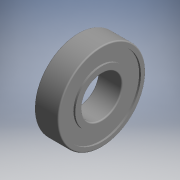
# Autodesk Inventor part: B6900ZZ
Saved by Autodesk Inventor 2017.3 (Build 213256000, 256)
## iProperties
Part Number: B6900ZZ
Material: Generic
Catalog Web Link: www.cadenas.de
Description: B6_ _ _ZZ, SB6_ _ _ZZ-Deep Groove Ball Bearings - Double Shield Type
Vendor: MISUMI
Document SubType Name: Modeling
Designer: partserver
Manufacturer: MISUMI
Mass: 1.66105 g
Surface Area: 12.7379 cm^2
Volume: 1.66105 cm^3
Density: 1 g/cm^3
Appearance: PSOLRGB-175-175-175
Category: PARTsolutions
Company: MISUMI
Title: B6900ZZ
Author: Cadenas PARTsolutions
Comments: Deep Groove Ball Bearings - Double Shield Type
PSOL_IDENT_0: {$CADENAS_DATA\23d-libs\misumi\metric\12_bearing_holders\sb6010zz.prj},171 {VTYP=3D},{NB=B6900ZZ},{L
PSOL_IDENT_1: INA=B6900ZZ},{NN=B6_ _ _ZZ, SB6_ _ _ZZ},{DATE=22.10.2019 07:39:52},{GEOMDATE=22.10.2019 06:26:04},{V
PSOL_IDENT_2: ERSION=},{LINEID=30},{WBVAR=TS},{WBNUMERIC=}  {NB=B6900ZZ},{LINA=B6900ZZ},{KT=DUMMY},{PN=B6900ZZ},{T
PSOL_IDENT_3: S=},{TS1= '', 'Steel', 'S', 'Stainless Steel'},{MAT=52100 Bearing Steel},{BN=6900ZZ},{DD=10},{D=22},
PSOL_IDENT_4: {B=6},{RR=0.3},{CR=2.70},{COR=1.27},{CRS=2.70},{CRSS=2.29},{CORS=1.27},{CORSS=1.02},{DD1=20.80},{R1=
PSOL_IDENT_5: 0.20},{R2=0.3},{DSMIN=12.0},{DSMAX=13.00},{DS1=13.00},{DDHH=20.0},{R=0.3},{MASS=9},{MASS11=9},{AA=5.
PSOL_IDENT_6: 1000},{BB=1.2000},{CC=1.7000},{TYS=w/o Retaining Ring}
NB: B6900ZZ
NN: B6_ _ _ZZ, SB6_ _ _ZZ
NT: Deep Groove Ball Bearings - Double Shield Type
NBSYN: $PN.
LINA: B6900ZZ
CATALOG: Misumi
PN: B6900ZZ
TS: Steel
MAT: 52100 Bearing Steel
BN: 6900ZZ
DD: 10
D: 22
B: 6
RR: 0.3
CR: 2.70
COR: 1.27
DSMIN: 12
DSMAX: 13
DDHH: 20
R: 0.3
MASS: 9
SUPPLIER: MISUMI
ARTICLENO: B6900ZZ
BOMINFO: B6900ZZ
CREATOR: CADENAS GmbH
Autodesk Inventor part; units mm, degrees
sketch "Sketch_1" plane through (0, 0, 0) normal (0, 0, 1) x (1, 0, 0)
  line L0 (6, 0) -> (0, 0)
  arc A0 (0, 5.3) -> (0.3, 5) centre (0.3, 5.3) ccw
  line L1 (0.3, 5) -> (5.7, 5)
  arc A1 (5.7, 5) -> (6, 5.3) centre (5.7, 5.3) ccw
  line L2 (6, 5.3) -> (6, 6.7)
  line L3 (6, 6.7) -> (5.55, 6.7)
  line L4 (5.55, 6.7) -> (5.55, 9.8)
  line L5 (5.55, 9.8) -> (6, 9.8)
  line L6 (6, 9.8) -> (6, 10.7)
  arc A2 (6, 10.7) -> (5.7, 11) centre (5.7, 10.7) ccw
  line L7 (5.7, 11) -> (0.3, 11)
  arc A3 (0.3, 11) -> (0, 10.7) centre (0.3, 10.7) ccw
  line L8 (0, 10.7) -> (0, 9.8)
  line L9 (0, 9.8) -> (0.45, 9.8)
  line L10 (0.45, 9.8) -> (0.45, 6.7)
  line L11 (0.45, 6.7) -> (0, 6.7)
  line L12 (0, 6.7) -> (0, 5.3)
  constraints: 26 end point, 8 point on circle, 4 centre point
revolve "Revolution1" add sketch "Sketch_1" angle 360 about axis through (6, 0, 0) along (1, 0, 0)
ref_plane "center_point_XY" through (3, 0, 0) normal (1, 0, 0) x (0, 0, -1)
ref_plane "center_point_YZ" through (3, 0, 0) normal (0, 0, -1) x (0, 1, 0)
ref_plane "center_point_ZX" through (3, 0, 0) normal (0, 1, 0) x (1, 0, 0)
ref_plane "to_housing_XY" through (0, 0, 0) normal (1, 0, 0) x (0, 0, -1)
ref_plane "to_housing_YZ" through (0, 0, 0) normal (0, 0, -1) x (0, 1, 0)
ref_plane "to_housing_ZX" through (0, 0, 0) normal (0, 1, 0) x (1, 0, 0)
ref_plane "to_ring_XY" through (5.1, 0, 0) normal (1, 0, 0) x (0, 0, -1)
ref_plane "to_ring_YZ" through (5.1, 0, 0) normal (0, 0, -1) x (0, 1, 0)
ref_plane "to_ring_ZX" through (5.1, 0, 0) normal (0, 1, 0) x (1, 0, 0)
body "Solid1"
